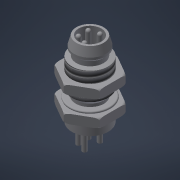
# Autodesk Inventor part: CH_0055_4_pin_connector
Saved by Autodesk Inventor 2022 (Build 260153000, 153)
## iProperties
Created: 2019-02-27
Part Number: CH_0055_4_pin_connector
Material: Generic
Document SubType Name: Modeling
Designer: Mario
Density: 1 g/cm^3
Appearance: Default
Author: Mario
Autodesk Inventor part; units mm, degrees
ref_plane "YZ Plane" through (0, 0, 0) normal (1, 0, 0) x (0, 1, 0)
ref_plane "XZ Plane" through (0, 0, 0) normal (0, 1, 0) x (-1, 0, 0)
ref_plane "XY Plane" through (0, 0, 0) normal (0, 0, 1) x (1, 0, 0)
sketch "Sketch1" plane through (0, 0, 0) normal (0, 1, 0) x (-1, 0, 0)
  line L0 (0, -5) -> (2.5, -5)
  line L1 (2.5, -5) -> (2.5, 0)
  line L2 (2.5, 0) -> (3, 0)
  line L3 (3, 0) -> (3.5, -1.866)
  line L4 (3.5, -1.866) -> (3.5, -2.366)
  line L5 (3.5, -2.366) -> (3, -2.866)
  line L6 (3, -2.866) -> (3, -3.866)
  line L7 (3, -3.866) -> (4, -4)
  line L8 (4, -4) -> (4, -10)
  line L9 (4, -10) -> (3, -11)
  line L10 (3, -11) -> (3, -12)
  line L11 (3, -12) -> (5.2735, -12)
  line L12 (5.7735, -12.5) -> (5.7735, -13.5)
  line L13 (5.2735, -14) -> (4, -14)
  line L14 (4, -14) -> (4, -16.5)
  line L15 (4, -16.5) -> (0, -16.5)
  line L16 (0, -16.5) -> (0, -5)
  line L17 (3, -11.75) -> (4.5, -11.75) construction
  line L18 (3.25, -11.5) -> (4.25, -11.5)
  line L19 (4.25, -12) -> (3.25, -12)
  arc A0 (3.25, -11.5) -> (3.25, -12) centre (3.25, -11.75) ccw
  arc A1 (4.25, -12) -> (4.25, -11.5) centre (4.25, -11.75) ccw
  line L20 (4, -8.5) -> (5.2735, -8.5)
  line L21 (5.7735, -8) -> (5.7735, -7)
  line L22 (5.2735, -6.5) -> (4, -6.5)
  line L23 (4, -6.5) -> (4, -8.5)
  arc A2 (5.7735, -7) -> (5.2735, -6.5) centre (5.2735, -7) ccw
  arc A3 (5.2735, -8.5) -> (5.7735, -8) centre (5.2735, -8) ccw
  arc A4 (5.7735, -12.5) -> (5.2735, -12) centre (5.2735, -12.5) ccw
  arc A5 (5.2735, -14) -> (5.7735, -13.5) centre (5.2735, -13.5) ccw
  point P0 (0, 0)
  point P1 (5.7735, -12)
  point P2 (5.7735, -14)
  point P3 (3.75, -11.75)
  point P4 (5.7735, -6.5)
  point P5 (5.7735, -8.5)
  dimension "d0" = 5
  dimension "d1" = 0
  dimension "d2" = 4
  dimension "d3" = 3.5
  dimension "d4" = 15
  dimension "d5" = 0.5
  dimension "d6" = 2.5
  dimension "d7" = 0.5
  dimension "d8" = 45
  dimension "d9" = 0
  dimension "d10" = 4
  dimension "d11" = 1
  dimension "d12" = 12
  dimension "d13" = 1
  dimension "d14" = 45
  dimension "d15" = 0
  dimension "d16" = 5.7735
  dimension "d17" = 0
  dimension "d18" = 2
  dimension "d19" = 16.5
  dimension "d20" = 0
  dimension "d43" = 1
  dimension "d44" = 0.25
  dimension "d45" = 0
  dimension "d46" = 2
  dimension "d47" = 0
  dimension "d48" = 3
  dimension "d49" = 0.5
  constraints: 50 end point, 14 point on circle, 12 point on line, 12 tangent, 7 perpendicular, 6 centre point, 5 horizontal, 5 parallel, 3 equal radius, 2 vertical, 1 midpoint
  measures "d0" distance from line of point (0, 0) L0
  measures "d1" vertical distance of point (0, 0) L1.end
  measures "d2" distance from line of point (0, 0) L8
  measures "d3" distance from line of point (0, 0) L4
  measures "d4" angle of L1 L3
  measures "d5" distance of L1.end L2.end
  measures "d6" distance from line of point (0, 0) L1
  measures "d7" distance of L3.end L4.end
  measures "d8" angle of L1 L5
  measures "d9" distance from line of L2.end L6
  measures "d10" distance from line of L7.end L2
  measures "d11" distance of L5.end L6.end
  measures "d12" distance from line of L11 point (0, 0)
  measures "d13" distance of L9.end L10.end
  measures "d14" angle of L10 L9
  measures "d15" distance between parallel lines of L6 L10
  measures "d16" horizontal distance of point (5.774, -12) point (0, 0)
  measures "d17" distance between parallel lines of L8 L14
  measures "d18" distance of point (5.774, -12) point (5.774, -14)
  measures "d19" vertical distance of L14.end point (0, 0)
  measures "d20" distance from line of point (0, 0) L16
  measures "d43" distance of L18.start L18.end
  measures "d44" radius of A1
  measures "d45" distance between parallel lines of L11 L19
  measures "d46" distance of point (5.774, -8.5) point (5.774, -6.5)
  measures "d47" distance between parallel lines of L12 L21
  measures "d48" distance between parallel lines of L20 L18
  measures "d49" radius of A2
revolve "Revolution1" add sketch "Sketch1" angle 360 about axis through (0, 0, -16.5) along (0, 0, 1) contours L0 L1 L2 L3 L4 L5 L6 L7 L8 L9 L10 L11 A4 L12 A5 L13 L14 L15 L16 | L11 A0 L18 A1 | L22 A2 L21 A3 L20 L8
sketch "Sketch2" plane through (0, 0, -12) normal (0, 0, 1) x (1, 0, 0)
  circle A0 centre (0, 0) radius 3 projected
  line L0 (-5, 2.8868) -> (0, 5.7735)
  line L1 (0, 5.7735) -> (5, 2.8868)
  line L2 (5, 2.8868) -> (5, -2.8868)
  line L3 (5, -2.8868) -> (0, -5.7735)
  line L4 (0, -5.7735) -> (-5, -2.8868)
  line L5 (-5, -2.8868) -> (-5, 2.8868)
  circle A1 centre (0, 0) radius 10.9
  point P0 (0, 0)
  dimension "d22" = 10
  dimension "d23" = 0
  constraints: 12 end point, 2 coincident, 1 centre point, 13 other
  measures "d22" distance between parallel lines of L3 L0
  measures "d23" horizontal distance of point (0, 0) L0.end
extrude "Extrusion1" cut sketch "Sketch2" along normal through all both and the other way through all contours A1
thread "Thread1" size "M8x1.25" class "6g" standard "ANSI Metric M Profile" full length
sketch "Sketch3" plane through (0, 0, 0) normal (0, 0, 1) x (1, 0, 0)
  circle A0 centre (0.5, 1.7) radius 0.5
  circle A1 centre (0.5, -1.7) radius 0.5
  circle A2 centre (-1.45, 1.075) radius 0.5
  circle A3 centre (-1.45, -1.075) radius 0.5
  point P0 (0, 0)
  dimension "d28" = 3.4
  dimension "d29" = 1.7
  dimension "d30" = 2.15
  dimension "d31" = 1.075
  dimension "d32" = 0
  dimension "d33" = 0
  dimension "d34" = 0.5
  dimension "d35" = 1.95
  dimension "d36" = 1
  dimension "d37" = 1
  dimension "d38" = 1
  dimension "d39" = 1
  constraints: 4 centre point
  measures "d28" distance of A1.centre A0.centre
  measures "d29" vertical distance of A0.centre point (0, 0)
  measures "d30" distance of A3.centre A2.centre
  measures "d31" vertical distance of point (0, 0) A2.centre
  measures "d32" horizontal distance of A3.centre A2.centre
  measures "d33" horizontal distance of A0.centre A1.centre
  measures "d34" horizontal distance of point (0, 0) A1.centre
  measures "d35" horizontal distance of A3.centre A1.centre
  measures "d36" diameter of A0
  measures "d37" diameter of A1
  measures "d38" diameter of A2
  measures "d39" diameter of A3
extrude "Extrusion2" add sketch "Sketch3" against normal blind 21
fillet "Fillet1" radius 0.5 4 edges at (-1.95, 1.075, 0) (0, 1.7, 0) (-1.95, -1.075, 0) (0, -1.7, 0)
equation "\"d46\" = d18"
equation "\"d29\" = 0.5 * d28"
equation "\"d31\" = 0.5 * d30"
equation "\"d37\" = d36"
equation "\"d38\" = d36"
equation "\"d39\" = d36"
body "Solid1"
